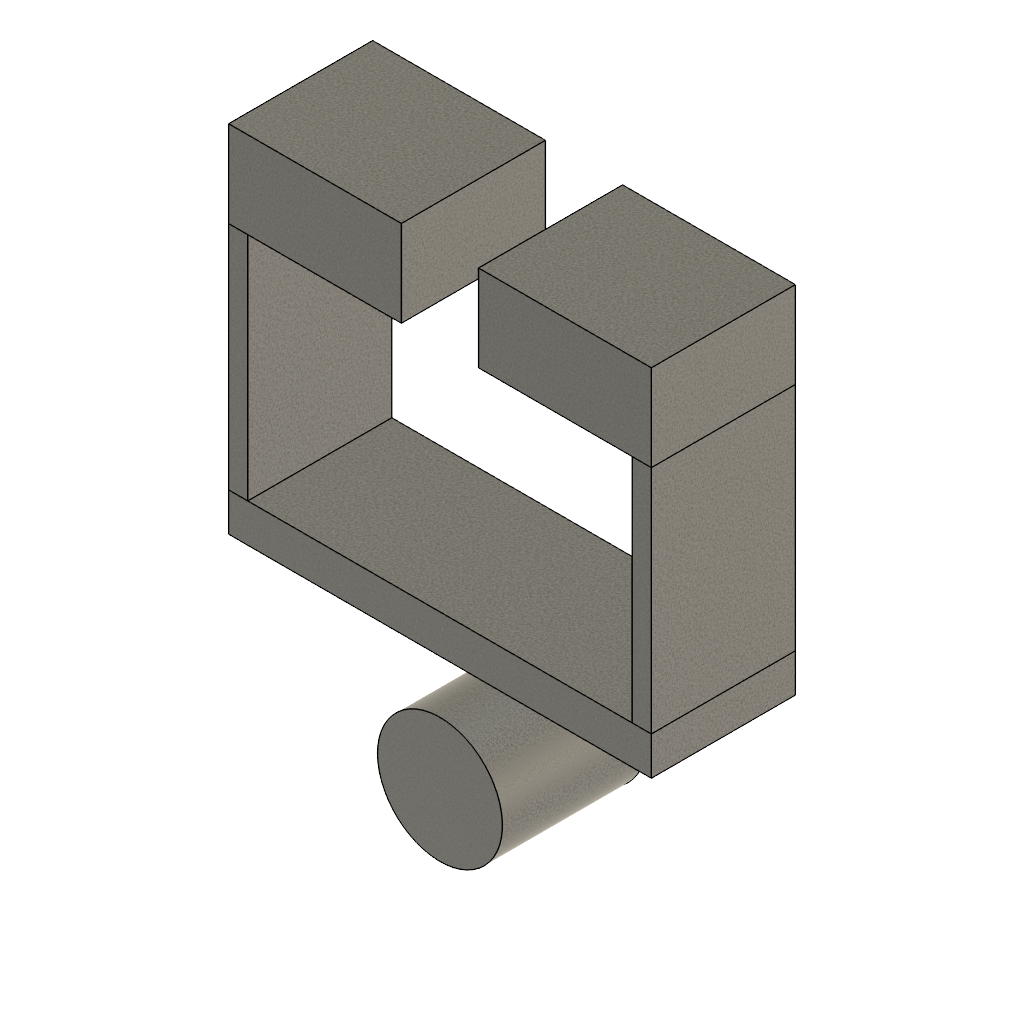
A6 (Autodesk Fusion 360 design; units mm, degrees)
part number: 2026-09-24-07-51-11-461
Autodesk Fusion 360 part; units mm, degrees
sketch "Sketch1" plane through (0, 0, 0) normal (0, 1, 0) x (1, 0, 0)
  circle A0 centre (0, 0) radius 10.3188
  dimension "d3" = 20.6375
  constraint coincident A0.centre origin
  measures "d3" diameter of A0
extrude "Extrude1" add sketch "Sketch1" along normal blind 23.8125 makes body 1
sketch "Sketch2" plane through (0, 23.8125, 0) normal (0, 1, 0) x (-1, 0, 0)
  circle A0 centre (0, 0) radius 10.3188
  line L0 (-10.3188, 0) -> (10.3188, 0)
  line L1 (10.3188, 0) -> (10.3188, 19.05)
  line L2 (10.3188, 19.05) -> (-10.3188, 19.05)
  line L3 (-10.3188, 19.05) -> (-10.3188, 0)
  dimension "d15" = 20.6375
  dimension "d16" = 19.05
  constraint horizontal L0
  constraint vertical L1
  constraint horizontal L2
  constraint vertical L3
  constraint coincident A0 L0.start
  measures "d15" distance of L0.start L0.end
  measures "d16" distance of L0.start L2.end
extrude "Extrude2" add sketch "Sketch2" against normal blind 4.7625 separate body contours A0 L1 L2 L3 makes body 2
sketch "Sketch3" plane through (0, 0, 19.05) normal (0, 0, 1) x (-1, 0, 0)
  line L0 (-10.3188, -23.8125) -> (10.3188, -23.8125)
  line L1 (10.3188, -23.8125) -> (10.3188, -19.05)
  line L2 (10.3188, -19.05) -> (-10.3188, -19.05)
  line L3 (-10.3188, -19.05) -> (-10.3188, -23.8125)
  line L4 (34.925, -23.8125) -> (-34.925, -23.8125)
  line L5 (-34.925, -23.8125) -> (-34.925, 0)
  line L6 (-34.925, 0) -> (34.925, 0)
  line L7 (34.925, 0) -> (34.925, -23.8125)
  dimension "d37" = 69.85
  dimension "d38" = 23.8125
  dimension "d39" = 34.925
  constraint horizontal L4
  constraint vertical L5
  constraint horizontal L6
  constraint vertical L7
  constraint coincident L0 L4.start
  measures "d37" distance of L4.start L4.end
  measures "d38" distance of L4.start L6.end
  measures "d39" distance of origin L5
extrude "Extrude5" add sketch "Sketch3" along normal blind 6.35 separate body makes body 3
sketch "Sketch4" plane through (0, 0, 25.4) normal (0, 0, 1) x (-1, 0, 0)
  line L0 (34.925, 0) -> (-34.925, 0)
  line L1 (-34.925, 0) -> (-34.925, -23.8125)
  line L2 (-34.925, -23.8125) -> (34.925, -23.8125)
  line L3 (34.925, -23.8125) -> (34.925, 0)
  line L4 (-34.925, 0) -> (-31.75, 0)
  line L5 (-31.75, 0) -> (-31.75, -23.8125)
  line L6 (-31.75, -23.8125) -> (-34.925, -23.8125)
  line L7 (-34.925, -23.8125) -> (-34.925, 0)
  line L8 (34.925, 0) -> (31.75, 0)
  line L9 (31.75, 0) -> (31.75, -23.8125)
  line L10 (31.75, -23.8125) -> (34.925, -23.8125)
  line L11 (34.925, -23.8125) -> (34.925, 0)
  dimension "d45" = 3.175
  dimension "d46" = 23.8125
  dimension "d47" = 3.175
  dimension "d48" = 23.8125
  constraint horizontal L4
  constraint vertical L5
  constraint horizontal L6
  constraint vertical L7
  constraint coincident L0.end L1.start
  constraint horizontal L8
  constraint vertical L9
  constraint horizontal L10
  constraint vertical L11
  constraint coincident L0.start L3.end
  measures "d45" distance of L0.end L4.end
  measures "d46" distance of L0.end L1.end
  measures "d47" distance of L0.start L8.end
  measures "d48" distance of L0.start L2.end
extrude "Extrude6" add sketch "Sketch4" along normal blind 38.1 separate body contours L0 L2 L3 L8 L9 L10 L11 | L0 L1 L2 L4 L5 L6 L7 makes body 4 at (-34.925, 15.875, 38.1) makes body 5 at (31.75, 7.9375, 38.1)
sketch "Sketch5" plane through (0, 0, 63.5) normal (0, 0, 1) x (-1, 0, 0)
  line L0 (-34.925, -23.8125) -> (-31.75, -23.8125)
  line L1 (-31.75, -23.8125) -> (-31.75, 0)
  line L2 (-31.75, 0) -> (-34.925, 0)
  line L3 (-34.925, 0) -> (-34.925, -23.8125)
  line L4 (-34.925, 0) -> (-6.3703, 0)
  line L5 (-6.3703, 0) -> (-6.3703, -23.8125)
  line L6 (-6.3703, -23.8125) -> (-34.925, -23.8125)
  line L7 (-34.925, -23.8125) -> (-34.925, 0)
  dimension "d54" = 28.5547
  dimension "d55" = 23.8125
  constraint horizontal L4
  constraint vertical L5
  constraint horizontal L6
  constraint vertical L7
  constraint coincident L2.end L3.start
  measures "d54" distance of L2.end L4.end
  measures "d55" distance of L2.end L0.start
sketch "Sketch6" plane through (0, 0, 63.5) normal (0, 0, 1) x (-1, 0, 0)
  line L0 (34.925, -23.8125) -> (34.925, 0)
  line L1 (34.925, 0) -> (31.75, 0)
  line L2 (31.75, 0) -> (31.75, -23.8125)
  line L3 (31.75, -23.8125) -> (34.925, -23.8125)
  line L4 (34.925, 0) -> (6.3703, 0)
  line L5 (6.3703, 0) -> (6.3703, -23.8125)
  line L6 (6.3703, -23.8125) -> (34.925, -23.8125)
  line L7 (34.925, -23.8125) -> (34.925, 0)
  dimension "d56" = 28.5547
  dimension "d57" = 23.8125
  constraint horizontal L4
  constraint vertical L5
  constraint horizontal L6
  constraint vertical L7
  constraint coincident L0.end L1.start
  measures "d56" distance of L0.end L4.end
  measures "d57" distance of L0.end L0.start
extrude "Extrude7" add sketch "Sketch5" sketch "Sketch6" along normal blind 14.2875 separate body of sketch 2 makes body 6 at (15.8885, 15.875, 63.5) makes body 7 at (-15.8885, 15.875, 63.5)
equation "D_A = 0.8125 in"
equation "L_A = 0.9375 in"
equation "d3 = D_A"
equation "d4 = L_A"
equation "b_B = D_A"
equation "L_B = 0.75 in"
equation "d15 = b_B"
equation "d16 = L_B"
equation "d17 = -H_B"
equation "L_C = L_A"
equation "d_C = 0.25 in"
equation "b_C = 2.75 in"
equation "d37 = b_C"
equation "d38 = L_C"
equation "d39 = b_C / 2"
equation "d40 = d_C"
equation "b_D = 0.125 in"
equation "d_D = 1.5 in"
equation "L_D = L_A"
equation "d45 = b_D"
equation "d46 = L_D"
equation "d47 = b_D"
equation "d48 = L_D"
equation "d49 = d_D"
equation "L_E = L_D"
equation "d_E = 0.5625 in"
equation "b_E = 1.1242 in"
equation "d54 = b_E"
equation "d55 = L_E"
equation "d56 = b_E"
equation "d57 = L_E"
equation "d58 = d_E"
equation "P = 1000 lbforce"
equation "stress = 9000 psi"
equation "H_B = ceil(( P / ( b_B * stress ) ) / 0.0625 in) * 0.0625 in"
named bodies: "Feature A", "Feature B", "Feature C", "Feature D_2", "Feature D_1", "Feature E_1", "Feature E_2"
